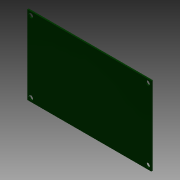
# Autodesk Inventor part: Parallella
Saved by Autodesk Inventor 2013 (Build 170138000, 138)
## iProperties
Created: 2014-04-13
Part Number: Parallella
Material: PCB(1)
Document SubType Name: Modeling
Designer: spichelh
Density: 1 g/cm^3
Author: spichelh
Autodesk Inventor part; units mm, degrees
ref_plane "YZ Plane" through (0, 0, 0) normal (1, 0, 0) x (0, 1, 0)
ref_plane "XZ Plane" through (0, 0, 0) normal (0, 1, 0) x (-1, 0, 0)
ref_plane "XY Plane" through (0, 0, 0) normal (0, 0, 1) x (1, 0, 0)
sketch "Sketch1" plane through (0, 0, 0) normal (0, 0, 1) x (1, 0, 0)
  line L0 (-43.18, -27.305) -> (43.18, -27.305)
  line L1 (43.18, -27.305) -> (43.18, 27.305)
  line L2 (43.18, 27.305) -> (-43.18, 27.305)
  line L3 (-43.18, 27.305) -> (-43.18, -27.305)
  line L4 (-43.18, -27.305) -> (43.18, 27.305) construction
  line L5 (43.18, -27.305) -> (-43.18, 27.305) construction
  circle A0 centre (-40.64, 24.765) radius 1.5
  line L6 (-43.18, 0) -> (43.18, 0) construction
  line L7 (0, 27.305) -> (0, -27.305) construction
  circle A1 centre (-40.64, -24.765) radius 1.5
  circle A2 centre (40.64, 24.765) radius 1.5
  circle A3 centre (40.64, -24.765) radius 1.5
  point P0 (0, 0)
  dimension "d2" = 86.36
  dimension "d4" = 54.61
  dimension "d6" = 3
  dimension "d21" = 2.54
  dimension "d22" = 2.54
  constraints: 16 end point, 6 midpoint, 4 centre point, 3 symmetric about line, 2 parallel, 1 horizontal, 1 perpendicular, 3 other
  measures "d2" distance of L1.end L2.end
  measures "d4" distance of L0.end L1.end
  measures "d6" diameter of A1
  measures "d21" distance from line of L1 A2.centre
  measures "d22" distance from line of L0 A1.centre
extrude "Extrusion1" add sketch "Sketch1" along normal blind 1
body "Solid1"
